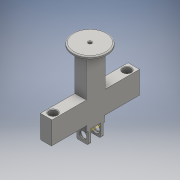
# Autodesk Inventor part: conductor
Saved by Autodesk Inventor 2016 (Build 200138000, 138)
## iProperties
Created: 2020-03-18
Part Number: conductor
Material: Genérico
Document SubType Name: Modeling
Designer: Andres Gomez
Density: 1 g/cm^3
Appearance: Valor por defecto
Author: Andres Gomez
Autodesk Inventor part; units mm, degrees
ref_plane "YZ Plane" through (0, 0, 0) normal (1, 0, 0) x (0, 1, 0)
ref_plane "XZ Plane" through (0, 0, 0) normal (0, 1, 0) x (-1, 0, 0)
ref_plane "XY Plane" through (0, 0, 0) normal (0, 0, 1) x (1, 0, 0)
ref_plane "Plano de trabajo1" through (0, 0, 2) normal (0, 0, 1) x (1, 0, 0)
sketch "Boceto1" plane through (0, 0, 2) normal (0, 0, 1) x (1, 0, 0)
  line L0 (-15.6511, 0) -> (-15.6511, 1)
  line L1 (-15.6511, 1) -> (-20.6511, 1)
  line L2 (-20.6511, 1) -> (-0.6511, 1)
  line L3 (-0.6511, 1) -> (-0.6511, 4)
  line L4 (-0.6511, 4) -> (-20.6511, 4)
  line L5 (-20.6511, 4) -> (-20.6511, 1)
  line L6 (-15.6511, -15.0414) -> (-15.6511, -16.0414)
  line L7 (-15.6511, -16.0414) -> (-20.6511, -16.0414)
  line L8 (-20.6511, -16.0414) -> (-20.6511, -19.0414)
  line L9 (-20.6511, -19.0414) -> (-0.6511, -19.0414)
  line L10 (-0.6511, -19.0414) -> (-0.6511, -16.0414)
  line L11 (-0.6511, -16.0414) -> (-15.6511, -16.0414)
  point P0 (0, 0)
  dimension "d0" = 1
  dimension "d1" = 5
  dimension "d2" = 20
  dimension "d3" = 3
  dimension "d4" = 1
  dimension "d5" = 5
  dimension "d6" = 3
  dimension "d7" = 20
  constraints: 24 end point, 8 point on line, 4 perpendicular, 1 vertical
  measures "d0" distance of L0.start L0.end
  measures "d1" distance of L0.end L1.end
  measures "d2" distance of L1.end L2.end
  measures "d3" distance of L2.end L3.end
  measures "d4" distance of L6.start L6.end
  measures "d5" distance of L6.end L7.end
  measures "d6" distance of L7.end L8.end
  measures "d7" distance of L8.end L9.end
extrude "Extrusión1" add sketch "Boceto1" against normal blind 20
sketch "Boceto2" plane through (0, 0, 2) normal (0, 0, 1) x (1, 0, 0)
  line L0 (-20.6511, -16.0414) -> (-20.6511, -19.0414) projected
  line L1 (-20.6511, -19.0414) -> (-20.6511, -24.0414)
  line L2 (-20.6511, -24.0414) -> (-0.6511, -24.0414)
  line L3 (-0.6511, 1) -> (-0.6511, 4) projected
  line L4 (-0.6511, -24.0414) -> (-0.6511, 4)
  line L5 (-0.6511, 4) -> (-0.6511, 9)
  line L6 (-0.6511, 9) -> (-20.6511, 9)
  line L7 (-20.6511, 9) -> (-20.6511, -19.0414)
  point P0 (0, 0)
  dimension "d11" = 5
  dimension "d12" = 20
  dimension "d13" = 5
  constraints: 12 end point, 2 perpendicular, 2 point on line, 1 collinear, 1 vertical
  measures "d11" distance of L0.end L1.end
  measures "d12" distance of L1.end L2.end
  measures "d13" distance of L3.end L5.end
extrude "Extrusión2" add sketch "Boceto2" along normal blind 120
sketch "Boceto3" plane through (0, 0, 122) normal (0, 0, 1) x (1, 0, 0)
  line L0 (-20.6511, -24.0414) -> (-0.6511, -24.0414) projected
  line L1 (-0.6511, 4) -> (-0.6511, 9) projected
  line L2 (-20.6511, -24.0414) -> (-0.6511, 9)
  line L3 (-0.6511, 9) -> (-20.6511, 9) projected
  line L4 (-20.6511, 9) -> (-0.6511, -24.0414)
  circle A0 centre (-10.6511, -7.5207) radius 30
  point P0 (0, 0)
  dimension "d16" = 60
  constraints: 4 end point, 1 centre point, 1 midpoint
  measures "d16" diameter of A0
extrude "Extrusión3" add sketch "Boceto3" along normal blind 4 contours L2 L4 L0 | L4 L3 L2 | A0
sketch "Boceto4" plane through (-20.6511, -24.0414, 2) normal (0, -1, 0) x (1, 0, 0)
  line L0 (20, 0) -> (0, 0) projected
  line L1 (10, 0) -> (10, 20)
  line L2 (20, 120) -> (0, 120) projected
  line L3 (10, 120) -> (10, 80)
  line L4 (20, 30) -> (0, 30)
  line L5 (0, 30) -> (0, 10)
  line L6 (0, 10) -> (20, 10)
  line L7 (20, 10) -> (20, 30)
  line L8 (20, 30) -> (0, 10) construction
  line L9 (0, 30) -> (20, 10) construction
  line L10 (20, 90) -> (0, 70) construction
  line L11 (0, 90) -> (20, 70) construction
  line L12 (0, 30) -> (20, 30)
  line L13 (20, 30) -> (20, 50)
  line L14 (20, 50) -> (0, 50)
  line L15 (0, 50) -> (0, 30)
  point P0 (20.6511, -2)
  dimension "d19" = 20
  dimension "d20" = 40
  dimension "d21" = 20
  dimension "d22" = 20
  dimension "d23" = 20
  dimension "d24" = 20
  dimension "d53" = 20
  dimension "d54" = 20
  constraints: 28 end point, 6 midpoint, 4 parallel, 2 horizontal, 2 perpendicular, 2 vertical
  measures "d19" distance of L1.start L1.end
  measures "d20" distance of L3.start L3.end
  measures "d21" distance of L6.end L5.end
  measures "d22" distance of L5.end L4.end
  measures "d23" distance of L11.end L10.end
  measures "d24" distance of L10.end L11.start
  measures "d53" distance of L14.end L13.end
  measures "d54" distance of L13.end L12.end
extrude "Extrusión4" add sketch "Boceto4" along normal blind 60
sketch "Boceto5" plane through (-20.6511, 9, 2) normal (0, 1, 0) x (1, 0, 0)
  line L0 (20, 0) -> (0, 0) projected
  line L1 (10, 0) -> (10, -20)
  line L2 (0, -120) -> (20, -120) projected
  line L3 (20, -90) -> (0, -70) construction
  line L4 (0, -90) -> (20, -70) construction
  line L5 (0, -10) -> (20, -10)
  line L6 (20, -10) -> (20, -30)
  line L7 (20, -30) -> (0, -30)
  line L8 (0, -30) -> (0, -10)
  line L9 (0, -10) -> (20, -30) construction
  line L10 (20, -10) -> (0, -30) construction
  line L11 (0, -30) -> (20, -30) projected
  line L12 (20, -30) -> (0, -30)
  line L13 (0, -30) -> (0, -50)
  line L14 (0, -50) -> (20, -50)
  line L15 (20, -50) -> (20, -30)
  point P0 (20.6511, 2)
  dimension "d27" = 20
  dimension "d29" = 20
  dimension "d30" = 20
  dimension "d31" = 20
  dimension "d32" = 20
  dimension "d50" = 20
  dimension "d51" = 20
  constraints: 26 end point, 4 parallel, 3 midpoint, 2 horizontal, 2 perpendicular, 1 vertical
  measures "d27" distance of L1.start L1.end
  measures "d29" distance of L3.end L4.end
  measures "d30" distance of L4.start L3.end
  measures "d31" distance of L6.end L7.end
  measures "d32" distance of L5.end L6.end
  measures "d50" distance of L14.end L13.end
  measures "d51" distance of L13.end L12.end
extrude "Extrusión5" add sketch "Boceto5" along normal blind 60
fillet "Empalme2" radius 1 4 edges at (-20.6511, -54.0414, 12) (-20.6511, 39, 12) (-0.6511, -54.0414, 12) (-0.6511, 39, 12)
sketch "Boceto8" plane through (-17.6511, -19.0414, -18) normal (0, -1, 0) x (1, 0, 0)
  circle A0 centre (7.8644, 10.8424) radius 6.2
  circle A1 centre (7.8644, 10.8424) radius 6.2
  point P0 (17.6511, 18)
  dimension "d42" = 12.4
  dimension "d64" = 12.4
  constraints: 2 centre point, 1 coincident
  measures "d42" diameter of A0
  measures "d64" diameter of A1
extrude "Extrusión7" cut sketch "Boceto8" against normal blind 30 and the other way blind 15
fillet "Empalme3" radius 2 2 edges at (-15.9867, -16.0414, -7.1576) (-15.9867, 1, -7.1576)
sketch "Boceto11" plane through (-1.6511, 9, 12) normal (0, 0, -1) x (-1, 0, 0)
  circle A0 centre (9, 48) radius 7 projected
  circle A1 centre (9, 48) radius 7
  circle A2 centre (9, -81.0677) radius 7
  point P0 (-1.6511, -9)
  dimension "d52" = 14
  constraints: 2 centre point, 1 coincident
  measures "d52" diameter of A2
extrude "Extrusión8" cut sketch "Boceto11" against normal blind 60
sketch "Boceto12" plane through (0, 0, 2) normal (0, 0, -1) x (-1, 0, 0)
  line L0 (0.6511, -19.0414) -> (1.6511, -19.0414) projected
  line L1 (0.6511, -19.0414) -> (20.6511, -19.0414)
  line L2 (20.6511, -19.0414) -> (20.6511, -20.5414)
  line L3 (20.6511, -20.5414) -> (0.6511, -20.5414)
  line L4 (0.6511, -20.5414) -> (0.6511, -19.0414)
  line L5 (0.6511, 9) -> (0.6511, 4) projected
  line L6 (20.6511, 9) -> (20.6511, -24.0414) projected
  line L7 (0.6511, 4) -> (20.6511, 4)
  line L8 (20.6511, 4) -> (20.6511, 5.5)
  line L9 (20.6511, 5.5) -> (0.6511, 5.5)
  line L10 (0.6511, 5.5) -> (0.6511, 4)
  point P0 (0, 0)
  dimension "d57" = 20
  dimension "d58" = 1.5
  dimension "d59" = 1.5
  constraints: 16 end point, 4 parallel, 2 horizontal, 2 perpendicular, 1 point on line
  measures "d57" distance of L2.end L3.end
  measures "d58" distance of L1.end L2.end
  measures "d59" distance of L8.end L7.end
extrude "Extrusión9" add sketch "Boceto12" along normal blind 20
sketch "Boceto13" plane through (-20.6511, 5.5, 2) normal (0, 1, 0) x (1, 0, 0)
  circle A0 centre (10.9301, 9.0935) radius 6.2
  point P0 (20.6511, 2)
  dimension "d65" = 12.4
  constraints: 1 centre point
  measures "d65" diameter of A0
extrude "Extrusión10" cut sketch "Boceto13" against normal blind 30
fillet "Empalme6" radius 2 4 edges at (-20.6511, 3.25, -18) (-20.6511, -18.2914, -18) (-0.6511, -18.2914, -18) (-0.6511, 3.25, -18)
sketch "Boceto14" plane through (-10.6511, -7.5207, 126) normal (0, 0, 1) x (1, 0, 0)
  circle A0 centre (0, 0) radius 2.5
  point P0 (10.6511, 7.5207)
  dimension "d69" = 5
  constraints: 1 centre point
  measures "d69" diameter of A0
extrude "Extrusión11" cut sketch "Boceto14" against normal blind 25
fillet "Empalme7" radius 1 1 edges at (-13.1511, -7.5207, 126)
fillet "Empalme8" radius 2 1 edges at (-40.6511, -7.5207, 126)
fillet "Empalme9" radius 1 4 edges at (-3.6511, -72.0677, 52) (-3.6511, 57, 52) (-3.6511, -72.0677, 12) (-3.6511, 57, 12)
fillet "Empalme11" radius 3 2 edges at (-20.6511, -7.5207, 2) (-0.6511, -7.5207, 2)
fillet "Empalme12" radius 1 10 edges at (-20.6511, -22.2914, 2) (-20.6511, -24.0414, 7.5) (-0.6511, -24.0414, 7.5) (-0.6511, -22.2914, 2) (-20.6511, 7.25, 2) (-0.6511, 7.25, 2) (-10.6511, 9, 2) (-20.6511, 9, 7.5) (-0.6511, 9, 7.5) (-10.6511, -24.0414, 2)
